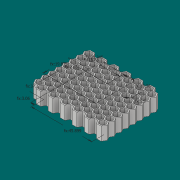
# Autodesk Inventor part: baffle
Saved by Autodesk Inventor 2021 (Build 250183000, 183)
## iProperties
Created: 2019-05-09
Part Number: baffle
Material: Generic
Document SubType Name: Modeling
Designer: uqspowe6
Density: 1 g/cm^3
Appearance: Default
Author: uqspowe6
Autodesk Inventor part; units mm, degrees
ref_plane "YZ Plane" through (0, 0, 0) normal (1, 0, 0) x (0, 1, 0)
ref_plane "XZ Plane" through (0, 0, 0) normal (0, 1, 0) x (-1, 0, 0)
ref_plane "XY Plane" through (0, 0, 0) normal (0, 0, 1) x (1, 0, 0)
sketch "Sketch1" plane through (0, 0, 0) normal (0, 1, 0) x (-1, 0, 0)
  line L0 (23.9456, -22.125) -> (22.6466, -19.875)
  line L1 (22.6466, -19.875) -> (23.9456, -17.625)
  line L2 (23.9456, -17.625) -> (26.5437, -17.625)
  line L3 (26.5437, -17.625) -> (27.8427, -19.875)
  line L4 (27.8427, -19.875) -> (26.5437, -22.125)
  line L5 (26.5437, -22.125) -> (23.9456, -22.125)
  line L6 (23.4837, -22.925) -> (21.9537, -20.275)
  line L7 (21.9537, -19.475) -> (23.2528, -17.225)
  line L8 (23.9456, -16.825) -> (27.0056, -16.825)
  line L9 (27.0056, -16.825) -> (28.7665, -19.875)
  line L10 (28.7665, -19.875) -> (27.0056, -22.925)
  line L11 (27.0056, -22.925) -> (23.4837, -22.925)
  line L12 (25.2446, -19.875) -> (20.6547, -19.875) construction
  line L13 (20.6547, -19.875) -> (20.6547, -17.225) construction
  line L14 (19.3557, -19.475) -> (18.0566, -17.225)
  line L15 (18.0566, -17.225) -> (19.3557, -14.975)
  line L16 (19.3557, -14.975) -> (21.9537, -14.975)
  line L17 (21.9537, -14.975) -> (23.2528, -17.225)
  line L18 (23.2528, -17.225) -> (21.9537, -19.475)
  line L19 (21.9537, -19.475) -> (19.3557, -19.475)
  line L20 (18.8938, -20.275) -> (17.1329, -17.225)
  line L21 (17.1329, -17.225) -> (18.8938, -14.175)
  line L22 (18.8938, -14.175) -> (22.4156, -14.175)
  line L23 (22.4156, -14.175) -> (23.9456, -16.825)
  line L24 (23.9456, -17.625) -> (22.6466, -19.875)
  line L25 (21.9537, -20.275) -> (18.8938, -20.275)
  line L26 (34.5198, 0) -> (-5.7533, 0) construction
  line L27 (0, -37.4544) -> (0, 8.2549) construction
  point P0 (20.6547, -19.475)
  dimension "d1" = 0.8
  dimension "d2" = 5.3
  dimension "d14" = 4.5899
  dimension "d15" = 2.65
  dimension "d16" = 0.8
  dimension "d17" = 5.3
  dimension "d42" = 0.8
  dimension "d43" = 0.8
  dimension "d44" = 0.8
  dimension "d45" = 0.8
  dimension "d46" = 19.875
  dimension "d47" = 25.2446
  constraints: 52 end point, 2 coincident, 1 horizontal, 1 midpoint, 1 perpendicular, 1 point on line, 30 other
  measures "d1" distance between parallel lines of L5 L11
  measures "d2" distance between parallel lines of L2 L11
  measures "d14" distance of L12.start L12.end
  measures "d15" distance of L12.end L13.end
  measures "d16" distance between parallel lines of L25 L19
  measures "d17" distance between parallel lines of L25 L16
  measures "d42" distance between parallel lines of L2 L8
  measures "d43" distance between parallel lines of L6 L0
  measures "d44" distance between parallel lines of L20 L14
  measures "d45" distance between parallel lines of L17 L23
  measures "d46" distance from line of L26 L12.start
  measures "d47" distance from line of L27 L12.start
extrude "Extrusion2" add sketch "Sketch1" along normal blind 10
pattern_linear "Rectangular Pattern3" count 2 spacing 9.1799 along (1, 0, 0) count 4 spacing 5.3 along (0, 0, 1) of "Extrusion2"
pattern_linear "Rectangular Pattern4" count 3 spacing 18.3597 along (1, 0, 0) count 2 spacing 21.2 along (0, 0, 1) of "Extrusion2", "Rectangular Pattern3"
sketch "Sketch4" plane through (0, 0, 0) normal (0, -1, 0) x (1, 0, 0)
  line L0 (9.9449, -17.225) -> (-8.4149, -17.225) construction
  line L1 (23.7147, 17.225) -> (-22.1847, 17.225) construction
  circle A0 centre (9.9449, -17.225) radius 0.75
  circle A1 centre (-8.4149, -17.225) radius 0.75
  circle A2 centre (-22.1847, 17.225) radius 0.75
  circle A3 centre (23.7147, 17.225) radius 0.75
  point P0 (0, 0)
  point P1 (-25.2446, -19.875)
  dimension "d54" = 18.3597
  dimension "d55" = 19.875
  dimension "d56" = 25.2446
  dimension "d57" = 16.8298
  dimension "d58" = 2.65
  dimension "d59" = 37.1
  dimension "d60" = 3.06
  dimension "d61" = 45.8993
  dimension "d79" = 1.5
  constraints: 4 centre point, 4 coincident, 4 end point, 3 equal radius, 2 horizontal
  measures "d54" distance of L0.start L0.end
  measures "d55" vertical distance of point (-25.245, -19.875) point (0, 0)
  measures "d56" horizontal distance of point (0, 0) point (-25.245, -19.875)
  measures "d57" horizontal distance of point (-25.245, -19.875) L0.end
  measures "d58" vertical distance of point (-25.245, -19.875) L0.end
  measures "d59" vertical distance of L1.end point (-25.245, -19.875)
  measures "d60" horizontal distance of L1.end point (-25.245, -19.875)
  measures "d61" distance of L1.start L1.end
  measures "d79" diameter of A0
extrude "Extrusion4" cut sketch "Sketch4" against normal blind 5
equation "\"origin_y\" = 19.875"
equation "\"origin_x\" = 25.24464"
equation "\"pitch\" = 5.3"
equation "\"wall_thickness\" = 0.8"
equation "\"pitch_x\" = 4.58993"
equation "\"cell_w\" = 6.11991"
equation "\"peg_dia\" = 1.5"
equation "\"peg_depth\" = 5"
equation "\"tab_width\" = 1"
equation "\"tab_height\" = 0.5"
equation "\"standoff\" = 1"
body "Solid2"
